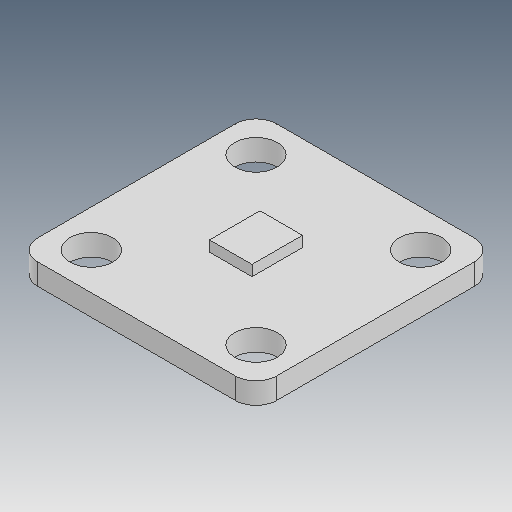
# Autodesk Inventor part: as5600
Saved by Autodesk Inventor 2025.2 (Build 292293000, 293)
## iProperties
Created: 2024-11-28
Part Number: as5600
Material: Generic
Document SubType Name: Modeling
Designer: email
Density: 1 g/cm^3
Appearance: Default
Author: email
Autodesk Inventor part; units mm, degrees
ref_plane "YZ Plane" through (0, 0, 0) normal (1, 0, 0) x (0, 1, 0)
ref_plane "XZ Plane" through (0, 0, 0) normal (0, 1, 0) x (-1, 0, 0)
ref_plane "XY Plane" through (0, 0, 0) normal (0, 0, 1) x (1, 0, 0)
sketch "Sketch1" plane through (0, 0, 0) normal (0, 1, 0) x (-1, 0, 0)
  line L0 (0, 0) -> (-22.86, 0)
  line L1 (-22.86, 0) -> (-22.86, -22.86)
  line L2 (-22.86, -22.86) -> (0, -22.86)
  line L3 (0, -22.86) -> (0, 0)
  line L4 (-22.86, -22.86) -> (-19.304, -22.86)
  line L5 (-19.304, -22.86) -> (-19.304, -19.304) construction
  line L6 (-19.304, -19.304) -> (-22.86, -19.304) construction
  line L7 (-22.86, -19.304) -> (-22.86, -22.86)
  line L8 (0, -22.86) -> (-3.556, -22.86)
  line L9 (-3.556, -22.86) -> (-3.556, -19.304) construction
  line L10 (-3.556, -19.304) -> (0, -19.304) construction
  line L11 (0, -19.304) -> (0, -22.86)
  line L12 (0, 0) -> (-3.556, 0)
  line L13 (-3.556, 0) -> (-3.556, -3.556) construction
  line L14 (-3.556, -3.556) -> (0, -3.556) construction
  line L15 (0, -3.556) -> (0, 0)
  line L16 (-22.86, 0) -> (-19.304, 0)
  line L17 (-19.304, 0) -> (-19.304, -3.556) construction
  line L18 (-19.304, -3.556) -> (-22.86, -3.556) construction
  line L19 (-22.86, -3.556) -> (-22.86, 0)
  circle A0 centre (-3.556, -19.304) radius 2.032
  circle A1 centre (-19.304, -19.304) radius 2.032
  circle A2 centre (-19.304, -3.556) radius 2.032
  circle A3 centre (-3.556, -3.556) radius 2.032
  line L20 (-3.556, -19.304) -> (-19.304, -19.304)
  line L21 (-19.304, -19.304) -> (-19.304, -3.556)
  line L22 (-19.304, -3.556) -> (-3.556, -3.556)
  line L23 (-3.556, -3.556) -> (-3.556, -19.304)
  dimension "d0" = 22.86
  dimension "d1" = 22.86
  dimension "d2" = 3.556
  dimension "d3" = 3.556
  dimension "d4" = 3.556
  dimension "d5" = 3.556
  dimension "d6" = 3.556
  dimension "d7" = 3.556
  dimension "d8" = 3.556
  dimension "d9" = 3.556
  dimension "d10" = 4.064
  dimension "d11" = 4.064
  dimension "d12" = 4.064
  dimension "d13" = 4.064
  constraints: 48 end point, 12 parallel, 6 horizontal, 6 perpendicular, 4 centre point, 4 coincident, 1 point on line
  measures "d0" distance of L1.end L2.end
  measures "d1" distance of L0.end L1.end
  measures "d2" distance of L8.end L9.end
  measures "d3" distance of L9.end L10.end
  measures "d4" distance of L13.end L14.end
  measures "d5" distance of L12.end L13.end
  measures "d6" distance of L17.end L18.end
  measures "d7" distance of L16.end L17.end
  measures "d8" distance of L5.end L6.end
  measures "d9" distance of L4.end L5.end
  measures "d10" diameter of A0
  measures "d11" diameter of A1
  measures "d12" diameter of A2
  measures "d13" diameter of A3
extrude "Extrusion1" add sketch "Sketch1" along normal blind 2.032 contours L3 L2 L1 L0 | A0 L20 A1 L21 A2 L22 A3 L23
fillet "Fillet1" radius 2 4 edges at (0, 1.016, 0) (22.86, 1.016, 0) (22.86, 1.016, -22.86) (0, 1.016, -22.86)
sketch "Sketch2" plane through (0, 2.032, 0) normal (0, 1, 0) x (1, 0, 0)
  line L0 (9.398, 13.843) -> (13.462, 13.843)
  line L1 (13.462, 13.843) -> (13.462, 9.017)
  line L2 (13.462, 9.017) -> (9.398, 9.017)
  line L3 (9.398, 9.017) -> (9.398, 13.843)
  line L4 (9.398, 13.843) -> (13.462, 9.017) construction
  line L5 (13.462, 13.843) -> (9.398, 9.017) construction
  line L6 (22.86, 2) -> (22.86, 20.86) projected
  line L7 (20.86, 22.86) -> (2, 22.86) projected
  point P0 (0, 0)
  point P1 (11.43, 11.43)
  dimension "d17" = 4.064
  dimension "d18" = 4.826
  dimension "d19" = 11.43
  dimension "d20" = 11.43
  constraints: 12 end point, 2 midpoint, 2 parallel, 1 horizontal, 1 perpendicular
  measures "d17" distance of L0.start L0.end
  measures "d18" distance of L0.end L1.end
  measures "d19" distance from line of L6 point (11.43, 11.43)
  measures "d20" distance from line of L7 point (11.43, 11.43)
extrude "Extrusion2" add sketch "Sketch2" along normal blind 1.016
body "Solid1"
